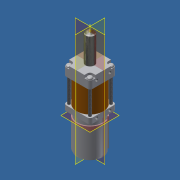
# Autodesk Inventor part: banebots_P6_3_stages
Saved by Autodesk Inventor 2016 (Build 200138000, 138)
## iProperties
Created: 2015-01-06
Part Number: banebots_P6_3_stages
Material: Aluminium 6061
Document SubType Name: Modeling
Designer: 4ndreas
Density: 2.71 g/cm^3
Appearance: Aluminium - flach
Author: 4ndreas
Autodesk Inventor part; units mm, degrees
ref_plane "YZ Plane" through (0, 0, 0) normal (1, 0, 0) x (0, 1, 0)
ref_plane "XZ Plane" through (0, 0, 0) normal (0, 1, 0) x (-1, 0, 0)
ref_plane "XY Plane" through (0, 0, 0) normal (0, 0, 1) x (1, 0, 0)
sketch "Skizze1" plane through (0, 0, 0) normal (0, 0, 1) x (1, 0, 0)
  line L0 (-19.05, 19.05) -> (19.05, 19.05)
  line L1 (19.05, 19.05) -> (19.05, -19.05)
  line L2 (19.05, -19.05) -> (-19.05, -19.05)
  line L3 (-19.05, -19.05) -> (-19.05, 19.05)
  line L4 (19.05, 19.05) -> (-19.05, -19.05) construction
  line L5 (-19.05, 19.05) -> (19.05, -19.05) construction
  point P0 (0, 0)
  point P1 (0, 0)
  dimension "d0" = 38.1
  constraints: 12 end point, 3 perpendicular, 2 midpoint, 2 parallel, 1 coincident, 1 horizontal
  measures "d0" distance between parallel lines of L1 L3
extrude "Extrusion1" add sketch "Skizze1" along normal blind 7.62
sketch "Skizze2" plane through (0, 0, 7.62) normal (0, 0, 1) x (1, 0, 0)
  line L0 (19.05, 19.05) -> (-19.05, 19.05) projected
  circle A0 centre (0, 0) radius 19.05
  constraints: 1 centre point, 1 coincident, 1 tangent
extrude "Extrusion2" add sketch "Skizze2" along normal blind 35.56
sketch "Skizze3" plane through (0, 0, 43.18) normal (0, 0, 1) x (1, 0, 0)
  line L0 (-19.05, 19.05) -> (19.05, 19.05) projected
  line L1 (19.05, 19.05) -> (19.05, -19.05) projected
  line L2 (19.05, -19.05) -> (-19.05, -19.05) projected
  line L3 (-19.05, -19.05) -> (-19.05, 19.05) projected
extrude "Extrusion3" add sketch "Skizze3" along normal blind 15.24
sketch "Skizze4" plane through (0, 0, 58.42) normal (0, 0, 1) x (1, 0, 0)
  circle A0 centre (0, 0) radius 6.35
  dimension "d7" = 12.7
  constraints: 1 centre point, 1 coincident
  measures "d7" diameter of A0
extrude "Extrusion4" add sketch "Skizze4" along normal blind 38.1
chamfer "Fase1" distance 1 angle 45 1 edges at (-6.35, 0, 96.52)
sketch "Skizze6" plane through (19.05, -19.05, 0) normal (1, 0, 0) x (0, 0, -1)
  line L0 (0, 38.1) -> (-7.62, 38.1) projected
  line L1 (0, 0) -> (-7.62, 0) projected
  line L2 (-43.18, 38.1) -> (-43.18, 19.05) projected
  line L3 (-43.18, 38.1) -> (-58.42, 38.1) projected
  line L4 (-58.42, 0) -> (-58.42, 38.1) projected
  line L5 (-43.18, 0) -> (-58.42, 0) projected
  line L6 (-43.18, 19.05) -> (-43.18, 0) projected
  line L7 (-50.8, 28.575) -> (-3.81, 28.575) construction
  line L8 (-3.81, 28.575) -> (-3.81, 9.525) construction
  line L9 (-3.81, 9.525) -> (-50.8, 9.525) construction
  line L10 (-50.8, 9.525) -> (-50.8, 28.575) construction
  line L11 (-43.18, 19.05) -> (-7.62, 19.05) construction
  line L12 (-3.81, 38.1) -> (-3.81, 0) construction
  point P0 (0, 19.05)
  dimension "d13" = 7.62
  dimension "d14" = 9.525
  constraints: 12 end point, 2 midpoint, 2 parallel, 2 perpendicular, 1 coincident, 1 collinear, 1 horizontal, 1 other
  measures "d13" distance between parallel lines of L10 L2
  measures "d14" distance between parallel lines of L11 L7
hole "Bohrung1" at (19.05, -9.525, 3.81) at (19.05, 9.525, 3.81) at (19.05, 9.525, 50.8) at (19.05, -9.525, 50.8) direction (-1, 0, 0) diameter 3.962 depth 8 tip angle 118 thread size "10-32 UNF" class "2B" standard "ANSI Unified Screw Threads"
fillet "Rundung1" radius 4 8 edges at (19.05, 19.05, 3.81) (-19.05, 19.05, 3.81) (19.05, -19.05, 3.81) (19.05, 19.05, 50.8) (19.05, -19.05, 50.8) (-19.05, 19.05, 50.8) (-19.05, -19.05, 50.8) (-19.05, -19.05, 3.81)
sketch "Skizze7" plane through (0, 0, 58.42) normal (0, 0, 1) x (1, 0, 0)
  line L0 (15.05, 19.05) -> (-15.05, 19.05) projected
  arc A0 (-15.05, 19.05) -> (-19.05, 15.05) centre (-15.05, 15.05) ccw projected
  line L1 (-19.05, 15.05) -> (-19.05, -15.05) projected
  arc A1 (-15.05, 11.05) -> (-11.05, 15.05) centre (-15.05, 15.05) ccw
  line L2 (-11.05, 15.05) -> (-11.05, 19.05)
  line L3 (-15.05, 11.05) -> (-19.05, 11.05)
  constraints: 4 end point, 2 perpendicular, 2 point on circle, 2 point on line, 2 tangent, 1 centre point, 1 coincident, 1 concentric
extrude "Extrusion5" cut sketch "Skizze7" against normal blind 4
sketch "Skizze8" plane through (0, 0, 54.42) normal (0, 0, 1) x (1, 0, 0)
  arc A0 (-15.05, 11.05) -> (-11.05, 15.05) centre (-15.05, 15.05) ccw projected
  circle A1 centre (-15.05, 15.05) radius 2
  point P0 (0, 0)
  dimension "d25" = 4
  constraints: 1 centre point, 1 coincident
  measures "d25" diameter of A1
extrude "Extrusion6" add sketch "Skizze8" against normal up to surface (46.8 mm away)
thread "Gewinde1" size "M4x0.7" class "6g" standard "ANSI Metric M Profile" full length
sketch "Skizze9" plane through (0, 0, 54.42) normal (0, 0, 1) x (1, 0, 0)
  arc A0 (-15.05, 19.05) -> (-19.05, 15.05) centre (-15.05, 15.05) ccw projected
  arc A1 (-15.05, 11.05) -> (-11.05, 15.05) centre (-15.05, 15.05) ccw projected
  circle A2 centre (-15.05, 15.05) radius 3.6
  point P0 (0, 0)
  dimension "d30" = 0.4
  constraints: 1 centre point, 1 coincident
  measures "d30" radial gap between concentric circles of A0 A2
extrude "Extrusion7" add sketch "Skizze9" along normal blind 2.5
fillet "Rundung2" radius 2 1 edges at (-18.65, 15.05, 56.92)
pattern_circular "Runde Anordnung1" count 4 over 360 about axis through (0, 0, 7.62) along (0, 0, 1) of "Extrusion6", "Extrusion7", "Rundung2", "Extrusion5"
sketch "Skizze10" plane through (0, 0, 0) normal (0, 0, -1) x (-1, 0, 0)
  circle A0 centre (0, 0) radius 17.907
  dimension "d37" = 35.814
  constraints: 1 centre point, 1 coincident
  measures "d37" diameter of A0
extrude "Extrusion8" add sketch "Skizze10" along normal blind 50
ref_plane "Arbeitsebene1" through (0, 0, -7) normal (0, 0, -1) x (-1, 0, 0)
sketch "Skizze11" plane through (0, 0, -7) normal (0, 0, -1) x (-1, 0, 0)
  arc A0 (-16.545, 6.8501) -> (-13.4778, 11.7903) centre (0, 0) ccw
  circle A1 centre (0, 0) radius 17.907 construction
  arc A2 (-17.8357, 7.3845) -> (-14.5292, 12.7101) centre (0, 0) ccw
  line L0 (-13.4778, 11.7903) -> (-14.5292, 12.7101)
  line L1 (-17.8357, 7.3845) -> (-16.545, 6.8501)
  dimension "d42" = 19.304
  constraints: 5 point on circle, 4 end point, 2 centre point, 2 coincident, 2 line through centre, 1 concentric
  measures "d42" radius of A2
extrude "Extrusion9" add sketch "Skizze11" along normal blind 40
ref_plane "Arbeitsebene2" through (0, 0, 7.62) normal (0, 1, 0) x (0, 0, 1)
ref_plane "Arbeitsebene3" through (0, 0, 7.62) normal (1, 0, 0) x (0, 0, 1)
mirror "Spiegeln1" about plane through (0, 0, 7.62) normal (1, 0, 0) of "Bohrung1"
